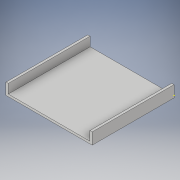
# Autodesk Inventor part: MAN_SERVO_HANDLER
Saved by Autodesk Inventor 2019 (Build 230136000, 136)
## iProperties
Created: 2021-03-07
Part Number: MAN_SERVO_HANDLER
Material: Generic
Document SubType Name: Modeling
Designer: DOMEK
Density: 1 g/cm^3
Appearance: Default
Author: DOMEK
Autodesk Inventor part; units mm, degrees
ref_plane "YZ Plane" through (0, 0, 0) normal (1, 0, 0) x (0, 1, 0)
ref_plane "XZ Plane" through (0, 0, 0) normal (0, 1, 0) x (-1, 0, 0)
ref_plane "XY Plane" through (0, 0, 0) normal (0, 0, 1) x (1, 0, 0)
sketch "Sketch2" plane through (0, 0, 0) normal (0, 1, 0) x (-1, 0, 0)
  line L0 (0, 0) -> (37.5, 0)
  line L1 (37.5, 0) -> (37.5, 35.6)
  line L2 (37.5, 35.6) -> (0, 35.6)
  line L3 (0, 35.6) -> (0, 0)
  dimension "d0" = 37.5
  dimension "d1" = 35.6
  constraints: 8 end point, 2 parallel, 1 horizontal, 1 perpendicular
  measures "d0" distance of L2.end L1.end
  measures "d1" distance of L1.end L0.end
extrude "Extrusion1" add sketch "Sketch2" along normal blind 1
sketch "Sketch4" plane through (0, 1, 0) normal (0, 1, 0) x (1, 0, 0)
  point P0 (0, 0)
sketch "Sketch5" plane through (0, 1, 0) normal (0, 1, 0) x (1, 0, 0)
  line L0 (-37.5, 0) -> (-37.5, -35.6) projected
  line L1 (-37.5, -35.6) -> (0, -35.6) projected
  line L2 (-37.5, 0) -> (-36.5, 0)
  line L3 (-36.5, 0) -> (-36.5, -35.6)
  line L4 (-36.5, -35.6) -> (-37.5, -35.6)
  line L5 (-37.5, -35.6) -> (-37.5, 0)
  line L6 (0, 0) -> (-37.5, 0) projected
  line L7 (0, 0) -> (-1, 0)
  line L8 (-1, 0) -> (-1, -35.6)
  line L9 (-1, -35.6) -> (0, -35.6)
  line L10 (0, -35.6) -> (0, 0)
  dimension "d6" = 1
  dimension "d7" = 1
  constraints: 16 end point, 4 parallel, 2 horizontal, 2 perpendicular, 2 point on line
  measures "d6" distance of L3.end L4.end
  measures "d7" distance of L9.end L8.end
extrude "Extrusion2" add sketch "Sketch5" along normal blind 4 contours L2 L3 L1 L0 | L6 L10 L1 L8
body "Solid1"
